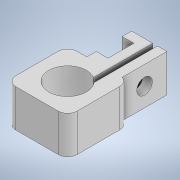
# Autodesk Inventor part: COLLIER
Saved by Autodesk Inventor 2020 (Build 240168000, 168)
## iProperties
Created: 2020-06-15
Part Number: COLLIER
Material: Generic
Document SubType Name: Modeling
Designer: Admin
Density: 1 g/cm^3
Appearance: Default
Author: Admin
Autodesk Inventor part; units mm, degrees
ref_plane "YZ Plane" through (0, 0, 0) normal (1, 0, 0) x (0, 1, 0)
ref_plane "XZ Plane" through (0, 0, 0) normal (0, 1, 0) x (-1, 0, 0)
ref_plane "XY Plane" through (0, 0, 0) normal (0, 0, 1) x (1, 0, 0)
sketch "Sketch4" plane through (0, 0, 0) normal (0, 1, 0) x (-1, 0, 0)
  line L0 (0, 0) -> (13, 0)
  line L1 (13, 0) -> (13, -13)
  line L2 (13, -13) -> (8.925, -13)
  line L3 (8.925, -13) -> (8.925, -22.5)
  line L4 (8.925, -22.5) -> (1.425, -22.5)
  line L5 (1.425, -22.5) -> (1.425, -13)
  line L6 (1.425, -13) -> (0, -13)
  line L7 (0, -13) -> (0, 0)
  dimension "d17" = 13
  dimension "d18" = 13
  dimension "d19" = 7.5
  dimension "d20" = 1.425
  dimension "d21" = 9.5
  constraints: 16 end point, 5 perpendicular, 2 horizontal, 2 point on line
  measures "d17" distance of L0.end L1.end
  measures "d18" distance of L0.start L0.end
  measures "d19" distance of L3.end L4.end
  measures "d20" distance of L5.end L6.end
  measures "d21" distance of L2.end L3.end
extrude "Extrusion2" add sketch "Sketch4" along normal blind 8
sketch "Sketch5" plane through (0, 8, 0) normal (0, 1, 0) x (1, 0, 0)
  line L0 (-8.925, 15) -> (-6.425, 15)
  line L1 (-6.425, 15) -> (-6.425, 20.5)
  line L2 (-6.425, 20.5) -> (-8.925, 20.5)
  line L3 (-8.925, 20.5) -> (-8.925, 15)
  line L4 (-1.425, 22.5) -> (-8.925, 22.5) projected
  line L5 (-8.925, 22.5) -> (-8.925, 13) projected
  point P0 (0, 0)
  dimension "d24" = 5.5
  dimension "d25" = 2.5
  dimension "d26" = 2
  constraints: 8 end point, 2 parallel, 1 horizontal, 1 perpendicular, 1 point on line
  measures "d24" distance of L2.end L0.start
  measures "d25" distance of L1.end L2.end
  measures "d26" distance between parallel lines of L4 L2
extrude "Extrusion3" cut sketch "Sketch5" against normal through all
sketch "Sketch6" plane through (0, 8, 0) normal (0, 1, 0) x (1, 0, 0)
  circle A0 centre (-6.5, 6.5) radius 4
  line L0 (-13, 0) -> (0, 0) projected
  line L1 (0, 0) -> (0, 13) projected
  dimension "d29" = 8
  dimension "d30" = 6.5
  dimension "d31" = 6.5
  constraints: 1 centre point
  measures "d29" diameter of A0
  measures "d30" distance from line of L0 A0.centre
  measures "d31" distance from line of L1 A0.centre
extrude "Extrusion4" cut sketch "Sketch6" against normal through all
sketch "Sketch7" plane through (0, 8, 0) normal (0, 1, 0) x (1, 0, 0)
  line L0 (-4.425, 8.5) -> (-3.425, 8.5)
  line L1 (-3.425, 8.5) -> (-3.425, 22.5)
  line L2 (-3.425, 22.5) -> (-4.425, 22.5)
  line L3 (-4.425, 22.5) -> (-4.425, 8.5)
  line L4 (-1.425, 22.5) -> (-8.925, 22.5) projected
  line L5 (-1.425, 13) -> (-1.425, 22.5) projected
  point P0 (0, 0)
  dimension "d34" = 1
  dimension "d35" = 14
  dimension "d36" = 2
  constraints: 8 end point, 2 parallel, 1 horizontal, 1 perpendicular, 1 point on line
  measures "d34" distance of L1.end L2.end
  measures "d35" distance of L2.end L0.start
  measures "d36" distance between parallel lines of L5 L1
extrude "Extrusion5" cut sketch "Sketch7" against normal through all
sketch "Sketch8" plane through (-1.425, 0, -13) normal (1, 0, 0) x (0, 0, -1)
  circle A0 centre (4.75, 4) radius 1.65
  line L0 (0, 0) -> (9.5, 0) projected
  line L1 (9.5, 0) -> (9.5, 8) projected
  point P0 (-13, 0)
  dimension "d39" = 3.3
  dimension "d40" = 4
  dimension "d41" = 4.75
  constraints: 1 centre point
  measures "d39" diameter of A0
  measures "d40" distance from line of A0.centre L0
  measures "d41" distance from line of A0.centre L1
extrude "Extrusion6" cut sketch "Sketch8" against normal through all
fillet "Fillet1" radius 2 4 edges at (-13, 4, -13) (-13, 4, 0) (0, 4, 0) (0, 4, -13)
body "Solid2"
